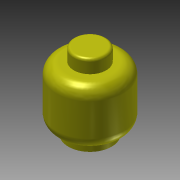
# Autodesk Inventor part: HEAD
Saved by Autodesk Inventor 2015 (Build 190159000, 159)
## iProperties
Created: 2012-05-01
Part Number: HEAD
Material: 250
Document SubType Name: Modeling
Mass: 5.11029 g
Surface Area: 4.75511 cm^2
Volume: 0.650992 cm^3
Density: 7.85 g/cm^3
Appearance: Steel
Autodesk Inventor part; units mm, degrees
ref_plane "YZ Plane" through (0, 0, 0) normal (1, 0, 0) x (0, 1, 0)
ref_plane "XZ Plane" through (0, 0, 0) normal (0, 1, 0) x (-1, 0, 0)
ref_plane "XY Plane" through (0, 0, 0) normal (0, 0, 1) x (1, 0, 0)
sketch "Sketch1" plane through (0, 0, 0) normal (0, 0, 1) x (1, 0, 0)
  line L0 (0, 5.785) -> (-2.44, 5.785)
  line L1 (-2.44, 5.785) -> (-2.44, 3.785)
  line L2 (-2.44, 3.785) -> (-5.055, 3.785)
  line L3 (-5.055, 3.785) -> (-5.055, -4.575)
  line L4 (-5.055, -4.575) -> (-3.26, -4.575)
  line L5 (-3.26, -4.575) -> (-3.26, -5.785)
  line L6 (-3.26, -5.785) -> (0, -5.785)
  line L7 (0, -5.785) -> (0, 5.785)
  point P0 (0, 0)
  point P1 (0, 0)
  dimension "d0" = 11.57
  dimension "d1" = 10.11
  dimension "d2" = 4.88
  dimension "d3" = 6.52
  dimension "d4" = 2
  dimension "d5" = 1.21
  constraints: 16 end point, 6 parallel, 1 coincident, 1 horizontal, 1 midpoint, 1 perpendicular
  measures "d0" distance between parallel lines of L6 L0
  measures "d1" diameter of L3 L7
  measures "d2" diameter of L1 L7
  measures "d3" diameter of L5 L7
  measures "d4" distance between parallel lines of L2 L0
  measures "d5" distance between parallel lines of L6 L4
revolve "Revolution1" add sketch "Sketch1" angle 360 about axis through (0, -5.785, 0) along (0, 1, 0)
fillet "Fillet1" radius 1.75 2 edges at (5.055, 3.785, 0) (5.055, -4.575, 0)
fillet "Fillet2" radius 0.4 1 edges at (2.44, 5.785, 0)
sketch "Sketch2" plane through (0, -5.785, 0) normal (0, -1, 0) x (1, 0, 0)
  circle A0 centre (0, 0) radius 3.26 projected
  circle A1 centre (0, 0) radius 2.5
  dimension "d9" = 5
  constraints: 1 centre point, 1 coincident
  measures "d9" diameter of A1
extrude "Extrusion1" cut sketch "Sketch2" against normal blind 3 contours A1
body "Solid1"
